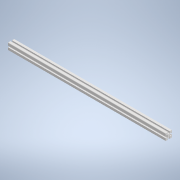
# Autodesk Inventor part: Extrusion
Saved by Autodesk Inventor 2020.2 (Build 242310000, 310)
## iProperties
Created: 2020-01-29
Part Number: Extrusion
Material: Generic
Document SubType Name: Modeling
Designer: Jimmy
Density: 1 g/cm^3
Appearance: Default
Author: Jimmy
Autodesk Inventor part; units mm, degrees
ref_plane "YZ Plane" through (0, 0, 0) normal (1, 0, 0) x (0, 1, 0)
ref_plane "XZ Plane" through (0, 0, 0) normal (0, 1, 0) x (-1, 0, 0)
ref_plane "XY Plane" through (0, 0, 0) normal (0, 0, 1) x (1, 0, 0)
sketch "Sketch2" plane through (0, 0, 0) normal (1, 0, 0) x (0, 1, 0)
  line L0 (1.3843, 0) -> (1.397, 0)
  line L1 (17.653, 0) -> (11.684, 0)
  line L2 (11.684, 0) -> (11.684, -1.397)
  line L3 (11.684, -1.397) -> (13.1572, -1.397)
  line L4 (13.1572, -1.397) -> (13.1572, -4.5085)
  line L5 (13.1572, -4.5085) -> (11.7024, -5.9633)
  line L6 (11.7024, -5.9633) -> (7.3844, -5.9633)
  line L7 (7.3844, -5.9633) -> (5.9296, -4.5085)
  line L8 (5.9296, -4.5085) -> (5.9296, -1.397)
  line L9 (5.9296, -1.397) -> (7.4028, -1.397)
  line L10 (7.4028, -1.397) -> (7.4028, 0)
  line L11 (1.397, 0) -> (7.4028, 0)
  line L12 (11.684, 0) -> (19.05, 0)
  line L13 (5.9633, -7.3476) -> (5.9633, -11.6656)
  line L14 (4.5085, -5.8928) -> (5.9633, -7.3476)
  line L15 (5.9633, -11.6656) -> (4.5085, -13.1204)
  line L16 (1.397, -13.1204) -> (1.397, -11.6472)
  line L17 (4.5085, -13.1204) -> (1.397, -13.1204)
  line L18 (1.397, -11.6472) -> (0, -11.6472)
  line L19 (1.397, -5.8928) -> (4.5085, -5.8928)
  line L20 (0, -7.366) -> (1.397, -7.366)
  line L21 (1.397, -7.366) -> (1.397, -5.8928)
  line L22 (7.3476, -13.0867) -> (11.6656, -13.0867)
  line L23 (5.8928, -14.5415) -> (7.3476, -13.0867)
  line L24 (11.6656, -13.0867) -> (13.1204, -14.5415)
  line L25 (13.1204, -17.653) -> (11.6472, -17.653)
  line L26 (13.1204, -14.5415) -> (13.1204, -17.653)
  line L27 (11.6472, -17.653) -> (11.6472, -19.05)
  line L28 (5.8928, -17.653) -> (5.8928, -14.5415)
  line L29 (7.366, -19.05) -> (7.366, -17.653)
  line L30 (7.366, -17.653) -> (5.8928, -17.653)
  line L31 (13.0867, -11.7024) -> (13.0867, -7.3844)
  line L32 (14.5415, -13.1572) -> (13.0867, -11.7024)
  line L33 (13.0867, -7.3844) -> (14.5415, -5.9296)
  line L34 (17.653, -5.9296) -> (17.653, -7.4028)
  line L35 (14.5415, -5.9296) -> (17.653, -5.9296)
  line L36 (17.653, -7.4028) -> (19.05, -7.4028)
  line L37 (17.653, -13.1572) -> (14.5415, -13.1572)
  line L38 (19.05, -11.684) -> (17.653, -11.684)
  line L39 (17.653, -11.684) -> (17.653, -13.1572)
  line L40 (1.3843, 0) -> (1.397, 0)
  line L41 (19.05, -1.397) -> (19.05, -7.4028)
  line L42 (19.05, -11.684) -> (19.05, -17.653)
  line L43 (17.653, -19.05) -> (11.6472, -19.05)
  line L44 (7.366, -19.05) -> (1.397, -19.05)
  line L45 (0, -17.653) -> (0, -11.6472)
  line L46 (0, -7.366) -> (0, -1.397)
  line L47 (0, -7.366) -> (0, -1.397)
  circle A0 centre (9.525, -9.525) radius 1.5875
  line L48 (1.3843, 0) -> (1.397, 0)
  line L49 (0, -1.397) -> (0, -1.3843)
  arc A1 (1.397, 0) -> (0, -1.397) centre (1.397, -1.397) ccw
  arc A2 (0, -17.653) -> (1.397, -19.05) centre (1.397, -17.653) ccw
  arc A3 (17.653, -19.05) -> (19.05, -17.653) centre (17.653, -17.653) ccw
  arc A4 (19.05, -1.397) -> (17.653, 0) centre (17.653, -1.397) ccw
  point P0 (0, 0)
  dimension "d34" = 7.366
  dimension "d35" = 1.397
  dimension "d37" = 1.4732
  dimension "d38" = 3.1115
  dimension "d39" = 2.0574
  dimension "d40" = 135
  dimension "d41" = 4.318
  dimension "d42" = 2.0574
  dimension "d43" = 1.4732
  dimension "d46" = 1.397
  dimension "d49" = 360
  dimension "d56" = 19.05
  dimension "d58" = 3.175
  dimension "d61" = 1.397
  dimension "d62" = 1.397
  dimension "d63" = 1.397
  dimension "d64" = 1.397
  dimension "d67" = 360
  dimension "d71" = 3.1115
  constraints: 100 end point, 11 perpendicular, 10 parallel, 8 point on circle, 5 centre point, 5 horizontal, 3 coincident, 2 point on line, 1 tangent, 96 other
  measures "d34" distance of L12.end L1.end
  measures "d35" distance of L1.end L2.end
  measures "d37" distance of L2.end L3.end
  measures "d38" distance of L3.end L4.end
  measures "d39" distance of L4.end L5.end
  measures "d40" angle of L4 L5
  measures "d41" distance of L5.end L6.end
  measures "d42" distance of L6.end L7.end
  measures "d43" distance of L8.end L9.end
  measures "d46" distance between parallel lines of L11 L9
  measures "d56" distance between parallel lines of L44 L11
  measures "d58" diameter of A0
  measures "d61" distance from line of L11 A1.centre
  measures "d62" distance from line of L46 A1.centre
  measures "d63" horizontal distance of point (0, 0) A1.centre
  measures "d64" horizontal distance of point (0, 0) A1.centre
  measures "d71" distance of L7.end L8.end
extrude "Extrusion1" add sketch "Sketch2" along normal blind 457.2
body "Solid1"
